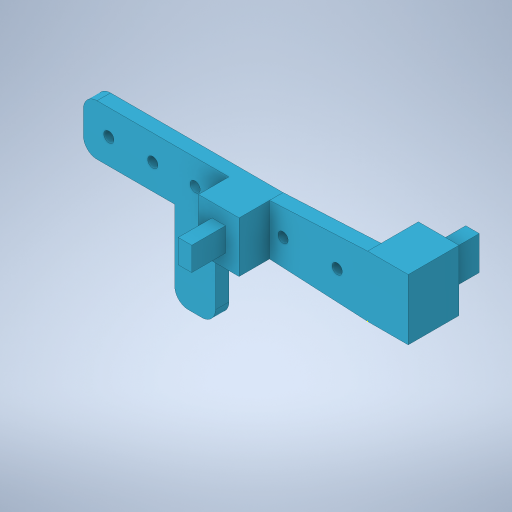
# Autodesk Inventor part: Mounting Bracket 3of4 - Copy
Saved by Autodesk Inventor 2024 (Build 280153000, 153)
## iProperties
Created: 2019-06-01
Part Number: Mounting Bracket 3of4 - Copy
Material: Generic
Document SubType Name: Modeling
Designer: cmcdona
Density: 1 g/cm^3
Appearance: Turquoise
Author: cmcdona
Autodesk Inventor part; units mm, degrees
ref_plane "YZ Plane" through (0, 0, 0) normal (1, 0, 0) x (0, 1, 0)
ref_plane "XZ Plane" through (0, 0, 0) normal (0, 1, 0) x (-1, 0, 0)
ref_plane "XY Plane" through (0, 0, 0) normal (0, 0, 1) x (1, 0, 0)
sketch "Sketch1" plane through (0, 0, 0) normal (0, 0, 1) x (1, 0, 0)
  line L0 (0, 0) -> (12, 0)
  line L1 (12, 0) -> (12, 18)
  line L2 (12, 18) -> (0, 18)
  line L3 (-29, 16.5) -> (-41, 16.5)
  line L4 (-41, 16.5) -> (-41, 1.5)
  line L5 (-41, 1.5) -> (-29, 1.5)
  line L6 (0, 18) -> (-29, 16.5)
  line L7 (0, 0) -> (-29, 1.5)
  circle A0 centre (-9, 9) radius 1.5
  dimension "d0" = 12
  dimension "d1" = 18
  dimension "d2" = 12
  dimension "d3" = 15
  dimension "d4" = 3
  constraints: 16 end point, 2 horizontal, 2 parallel, 2 perpendicular, 1 centre point
  measures "d0" distance of L2.end L1.end
  measures "d1" distance of L1.end L0.end
  measures "d2" distance of L5.end L4.end
  measures "d3" distance of L4.end L3.end
  measures "d4" diameter of A0
extrude "Extrusion1" add sketch "Sketch1" along normal blind 4
sketch "Sketch2" plane through (0, 0, 0) normal (0, 0, -1) x (-1, 0, 0)
  line L0 (0, 18) -> (29, 16.5) projected
  line L1 (0, 18) -> (-12, 18)
  line L2 (-12, 18) -> (-12, 0)
  line L3 (-12, 0) -> (0, 0)
  line L4 (0, 0) -> (0, 18)
  dimension "d11" = 12
  dimension "d7" = 12
  dimension "d8" = 18
  constraints: 8 end point, 2 parallel, 1 horizontal, 1 perpendicular
  measures "d7" distance of L3.end L2.end
  measures "d8" distance of L2.end L1.end
extrude "Extrusion2" add sketch "Sketch2" along normal blind 11
sketch "Sketch3" plane through (0, 0, 4) normal (0, 0, 1) x (1, 0, 0)
  line L0 (-29, 16.5) -> (-41, 16.5) projected
  line L1 (-41, 16.5) -> (-29, 16.5)
  line L2 (-29, 16.5) -> (-29, 1.5)
  line L3 (-29, 1.5) -> (-41, 1.5)
  line L4 (-41, 1.5) -> (-41, 16.5)
  point P0 (0, 0)
  dimension "d11" = 12
  dimension "d12" = 15
  constraints: 8 end point, 2 parallel, 1 horizontal, 1 perpendicular
  measures "d11" distance of L2.end L3.end
  measures "d12" distance of L1.end L2.end
extrude "Extrusion3" add sketch "Sketch3" along normal blind 9
sketch "Sketch4" plane through (0, 0, -11) normal (0, 0, -1) x (-1, 0, 0)
  line L0 (-4, 4) -> (-8, 4)
  line L1 (-8, 4) -> (-8, 14)
  line L2 (-8, 14) -> (-4, 14)
  line L3 (-4, 14) -> (-4, 4)
  point P0 (0, 0)
  dimension "d15" = 4
  dimension "d16" = 10
  constraints: 8 end point, 2 parallel, 1 horizontal, 1 perpendicular
  measures "d15" distance of L1.end L2.end
  measures "d16" distance of L0.end L1.end
extrude "Extrusion4" add sketch "Sketch4" along normal blind 10
sketch "Sketch5" plane through (0, 0, 13) normal (0, 0, 1) x (1, 0, 0)
  line L0 (-33, 5.5) -> (-37, 5.5)
  line L1 (-37, 5.5) -> (-37, 12.5)
  line L2 (-37, 12.5) -> (-33, 12.5)
  line L3 (-33, 12.5) -> (-33, 5.5)
  point P0 (0, 0)
  dimension "d19" = 4
  dimension "d20" = 7
  constraints: 8 end point, 2 parallel, 1 horizontal, 1 perpendicular
  measures "d19" distance of L1.end L2.end
  measures "d20" distance of L0.end L1.end
extrude "Extrusion5" add sketch "Sketch5" along normal blind 10
sketch "Sketch6" plane through (0, 0, 0) normal (0, 0, -1) x (-1, 0, 0)
  line L0 (41, 16.5) -> (41, 1.5)
  circle A0 centre (51, 9) radius 1.5
  line L1 (41, 16.5) -> (41, 1.5) projected
  line L2 (84, 1.5) -> (84, 16.5)
  line L3 (84, 16.5) -> (41, 16.5)
  line L4 (41, 16.5) -> (41, 1.5)
  line L5 (57, 1.5) -> (57, -23.5)
  line L6 (57, -23.5) -> (45, -23.5)
  line L7 (45, -23.5) -> (45, 1.5)
  line L8 (41, 1.5) -> (45, 1.5)
  line L9 (57, 1.5) -> (84, 1.5)
  point P0 (0, 0)
  dimension "d26" = 3
  dimension "d29" = 43
  dimension "d30" = 15
  dimension "d31" = 12
  dimension "d32" = 25
  dimension "d33" = 4
  constraints: 18 end point, 5 parallel, 2 horizontal, 2 perpendicular, 1 centre point
  measures "d26" diameter of A0
  measures "d29" distance of L3.end L2.end
  measures "d30" distance of L2.end L2.start
  measures "d31" distance of L5.end L6.end
  measures "d32" distance of L5.start L5.end
  measures "d33" distance of L0.end L7.end
extrude "Extrusion7" add sketch "Sketch6" against normal blind 4
fillet "Fillet2" radius 4 4 edges at (-84, 16.5, 2) (-84, 1.5, 2) (-57, -23.5, 2) (-45, -23.5, 2)
sketch "Sketch7" plane through (0, 0, 4) normal (0, 0, 1) x (1, 0, 0)
  circle A0 centre (-63.5, 9) radius 1.5
  circle A1 centre (-76.5, 9) radius 1.5
  line L0 (-29, 16.5) -> (-41, 16.5) projected
  circle A2 centre (-51, 9) radius 1.5 projected
  point P0 (0, 0)
  dimension "d39" = 3
  dimension "d40" = 3
  dimension "d41" = 7.5
  dimension "d42" = 7.5
  dimension "d43" = 12.5
  dimension "d44" = 13
  constraints: 2 centre point
  measures "d39" diameter of A0
  measures "d40" diameter of A1
  measures "d41" distance from line of L0 A0.centre
  measures "d42" distance from line of L0 A1.centre
  measures "d43" distance of A2.centre A0.centre
  measures "d44" distance of A1.centre A0.centre
extrude "Extrusion8" cut sketch "Sketch7" against normal through all contours A0 | A1
sketch "Sketch8" plane through (0, 0, 4) normal (0, 0, 1) x (1, 0, 0)
  circle A0 centre (-51, -7) radius 1.5
  line L0 (-45, -19.5) -> (-45, 1.5) projected
  circle A1 centre (-51, 9) radius 1.5 projected
  point P0 (0, 0)
  dimension "d47" = 3
  dimension "d48" = 6
  dimension "d49" = 16
  constraints: 1 centre point
  measures "d47" diameter of A0
  measures "d48" distance from line of A0.centre L0
  measures "d49" distance of A1.centre A0.centre
extrude "Extrusion9" cut sketch "Sketch8" against normal through all contours A0
sketch "Sketch9" plane through (0, 0, 4) normal (0, 0, 1) x (1, 0, 0)
  point P0 (0, 0)
sketch "Sketch10" plane through (0, 0, 4) normal (0, 0, 1) x (1, 0, 0)
  circle A0 centre (-25, 9) radius 1.5
  line L0 (-29, 16.5) -> (-41, 16.5) projected
  circle A1 centre (-9, 9) radius 1.5 projected
  point P0 (0, 0)
  dimension "d52" = 3
  dimension "d53" = 7.5
  dimension "d54" = 16
  constraints: 1 centre point
  measures "d52" diameter of A0
  measures "d53" distance from line of A0.centre L0
  measures "d54" distance of A0.centre A1.centre
extrude "Extrusion10" cut sketch "Sketch10" against normal through all contours A0
body "Solid1"
